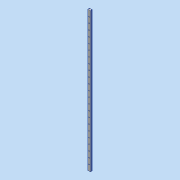
# Autodesk Inventor part: Prowadnica liniowa typu MGN12H 600mm
Saved by Autodesk Inventor 2018 (Build 220112000, 112)
## iProperties
Created: 2019-01-26
Part Number: Prowadnica liniowa typu MGN12H 600mm
Material: Ogólny
Document SubType Name: Modeling
Designer: Dawid
Density: 1 g/cm^3
Appearance: Aluminium — płaski
Author: Dawid
Autodesk Inventor part; units mm, degrees
ref_plane "YZ Plane" through (0, 0, 0) normal (1, 0, 0) x (0, 1, 0)
ref_plane "XZ Plane" through (0, 0, 0) normal (0, 1, 0) x (-1, 0, 0)
ref_plane "XY Plane" through (0, 0, 0) normal (0, 0, 1) x (1, 0, 0)
sketch "Szkic1" plane through (0, 0, 0) normal (0, 0, 1) x (1, 0, 0)
  line L0 (-6, -4) -> (6, -4)
  line L1 (6, 4) -> (-6, 4)
  line L2 (-6, 4) -> (-6, 2.5)
  line L3 (-6, 2.5) -> (-4.5, 2.5)
  line L4 (-4.5, 2.5) -> (-4.5, 1)
  line L5 (-4.5, 1) -> (-6, 1)
  line L6 (-6, 4) -> (-6, 2.5)
  line L7 (-6, 1) -> (-6, -4)
  line L8 (6, 4) -> (6, 2.5)
  line L9 (6, 2.5) -> (4.5, 2.5)
  line L10 (4.5, 2.5) -> (4.5, 1)
  line L11 (4.5, 1) -> (6, 1)
  line L12 (6, -4) -> (6, 1)
  line L13 (6, 2.5) -> (6, 4)
  point P0 (0, 0)
  dimension "d0" = 12
  dimension "d1" = 8
  constraints: 28 end point, 9 perpendicular, 5 parallel, 1 horizontal
  measures "d0" distance of L1.end L1.start
  measures "d1" distance of L1.start L0.end
extrude "Wyciągnięcie proste1" add sketch "Szkic1" along normal blind 600
sketch "Szkic2" plane through (-6, 4, 600) normal (0, 1, 0) x (1, 0, 0)
  line L0 (12, 600) -> (0, 600) projected
  line L1 (0, 600) -> (0, 0) projected
  line L2 (12, 0) -> (0, 0) projected
  line L3 (12, 600) -> (12, 0) projected
  line L4 (6, 600) -> (6, 0)
  line L5 (0, 0) -> (12, 0) projected
  line L6 (6, 0) -> (6, 25)
  circle A0 centre (6, 25) radius 1.75
  dimension "d10" = 25
  dimension "d11" = 3.5
  constraints: 4 end point, 1 centre point, 1 coincident, 1 midpoint, 1 point on line
  measures "d10" distance of L4.end L6.end
  measures "d11" diameter of A0
extrude "Wyciągnięcie proste2" cut sketch "Szkic2" against normal up to next contours A0 L4 | L4 A0
sketch "Szkic3" plane through (-6, 4, 600) normal (0, 1, 0) x (1, 0, 0)
  circle A0 centre (6, 25) radius 1.75 projected
  circle A1 centre (6, 25) radius 3
  point P0 (6, 600)
  dimension "d14" = 6
  constraints: 1 centre point, 1 coincident
  measures "d14" diameter of A1
extrude "Wyciągnięcie proste3" cut sketch "Szkic3" against normal blind 4.5
pattern_linear "Szyk prostokątny1" count 23 spacing 25 along (0, 0, -1) of "Wyciągnięcie proste2"
pattern_linear "Szyk prostokątny2" count 23 spacing 25 along (0, 0, -1) of "Wyciągnięcie proste3"
